Autodesk Fusion 360 part; units mm, degrees
(part 3 of 3)
equation "wall_thickness = 3 mm"
equation "d92 = wall_thickness"
equation "d94 = dowel_hole_diameter + 2 * dowel_hole_wall"
equation "d95 = dowel_hole_diameter + 2 * dowel_hole_wall"
equation "dowel_hole_height = 5 mm"
equation "d97 = dowel_hole_height + wall_thickness"
equation "d99 = wall_thickness"
equation "d130 = base_width"
equation "d134 = wall_thickness"
equation "d136 = wall_thickness"
equation "d137 = wall_thickness"
equation "d140 = wall_thickness"
equation "d146 = base_width"
equation "d149 = wall_thickness"
equation "d151 = wall_thickness"
equation "d152 = wall_thickness"
equation "d155 = wall_thickness"
equation "d157 = wall_thickness"
equation "d159 = thickness + 10 mm + 17.5 mm"
equation "d160 = 12 mm + slider_clearence"
equation "d162 = dowel_hole_wall"
equation "d163 = dowel_hole_wall"
equation "d169 = wall_thickness"
equation "backing_screw_hole_diam = 3 mm"
equation "d174 = peg_diameter + 0.3 mm"
equation "d175 = peg_diameter + 0.3 mm"
equation "d176 = -connector_thickness"
equation "d187 = cap_size"
equation "d188 = cap_size"
equation "cap_size = 6 mm"
named bodies: "Spur Gear (12 teeth)", "Connecting Rod", "Slider", "Base Plate", "Bottom Plate", "Side panel 1", "Side panel 2", "Top Plate", "Cap 1", "Cap 2"
